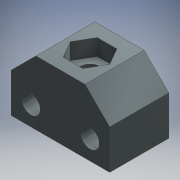
# Autodesk Inventor part: back_sprocket_holder
Saved by Autodesk Inventor 2016 (Build 200138000, 138)
## iProperties
Created: 2017-01-06
Part Number: back_sprocket_holder
Material: Generic
Document SubType Name: Modeling
Designer: hesaon
Density: 1 g/cm^3
Appearance: Default
Author: hesaon
Autodesk Inventor part; units mm, degrees
ref_plane "YZ Plane" through (0, 0, 0) normal (1, 0, 0) x (0, 1, 0)
ref_plane "XZ Plane" through (0, 0, 0) normal (0, 1, 0) x (-1, 0, 0)
ref_plane "XY Plane" through (0, 0, 0) normal (0, 0, 1) x (1, 0, 0)
sketch "Sketch1" plane through (0, 0, 0) normal (0, 1, 0) x (-1, 0, 0)
  line L0 (0, 0) -> (30, 0)
  line L1 (30, 0) -> (30, -12)
  line L2 (30, -12) -> (0, -12)
  line L3 (0, -12) -> (0, 0)
  circle A0 centre (24, -6) radius 2.85
  circle A1 centre (6, -6) radius 2.85
  dimension "d0" = 30
  dimension "d1" = 12
  dimension "d2" = 5.7
  dimension "d3" = 5.7
  dimension "d4" = 6
  dimension "d5" = 18
  dimension "d6" = 6
  constraints: 8 end point, 2 centre point, 2 parallel, 1 horizontal, 1 horizontal alignment, 1 perpendicular
  measures "d0" distance of L1.end L2.end
  measures "d1" distance of L0.end L1.end
  measures "d2" diameter of A0
  measures "d3" diameter of A1
  measures "d4" distance from line of L1 A0.centre
  measures "d5" distance of A1.centre A0.centre
  measures "d6" distance from line of L2 A0.centre
extrude "Extrusion1" add sketch "Sketch1" along normal blind 18
sketch "Sketch4" plane through (0, 0, -12) normal (0, 0, -1) x (-1, 0, 0)
  circle A0 centre (15, 9) radius 3
  line L0 (30, 0) -> (0, 0) projected
  line L1 (0, 0) -> (0, 18) projected
  dimension "d14" = 6
  dimension "d15" = 9
  dimension "d16" = 15
  constraints: 1 centre point
  measures "d14" diameter of A0
  measures "d15" distance from line of L0 A0.centre
  measures "d16" distance from line of L1 A0.centre
sketch "Sketch5" plane through (0, 0, 0) normal (0, -1, 0) x (1, 0, 0)
  line L0 (-30, 0) -> (-22.5, 7.5)
  line L1 (-22.5, 7.5) -> (-7.5, 7.5)
  line L2 (0, 0) -> (0, -12) projected
  line L3 (-7.5, 7.5) -> (0, 0)
  line L4 (0, 0) -> (-30, 0) projected
  line L5 (-30, 0) -> (0, 0) projected
  line L6 (-30, 0) -> (0, 0)
  dimension "d19" = 7.5
  dimension "d20" = 7.5
  dimension "d21" = 15
  dimension "d22" = 7.5
  dimension "d23" = 135
  constraints: 8 end point, 2 horizontal
  measures "d19" distance from line of L2 L1.end
  measures "d20" distance between parallel lines of L4 L1
  measures "d21" distance of L1.end L0.end
  measures "d22" horizontal distance of L0.start L0.end
  measures "d23" angle of L0 L1
extrude "Extrusion5" add sketch "Sketch5" against normal blind 18
extrude "Extrusion6" cut sketch "Sketch4" against normal through all
sketch "Sketch6" plane through (-22.5, 0, 7.5) normal (0, 0, 1) x (1, 0, 0)
  line L0 (1.4956, 9) -> (4.4978, 14.2)
  line L1 (4.4978, 14.2) -> (10.5022, 14.2)
  line L2 (10.5022, 14.2) -> (13.5044, 9)
  line L3 (13.5044, 9) -> (10.5022, 3.8)
  line L4 (10.5022, 3.8) -> (4.4978, 3.8)
  line L5 (4.4978, 3.8) -> (1.4956, 9)
  line L6 (0, 18) -> (15, 18) projected
  point P0 (22.5, 0)
  point P1 (7.5, 9)
  point P2 (7.5, 9)
  dimension "d30" = 10.4
  constraints: 12 end point, 1 coincident, 1 parallel, 13 other
  measures "d30" distance between parallel lines of L0 L3
extrude "Extrusion7" cut sketch "Sketch6" against normal blind 5
body "Solid1"
